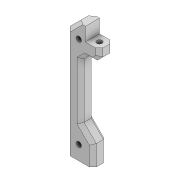
# Autodesk Inventor part: rackstand-v2-left
Saved by Autodesk Inventor 2020 (Build 240168000, 168)
## iProperties
Created: 2021-07-06
Part Number: rackstand-v2-left
Material: Generic
Document SubType Name: Modeling
Designer: Aidan Lee
Density: 1 g/cm^3
Appearance: Default
Author: Aidan Lee
Autodesk Inventor part; units mm, degrees
ref_plane "YZ Plane" through (0, 0, 0) normal (1, 0, 0) x (0, 1, 0)
sketch "Sketch1" plane through (0, 0, 0) normal (0, 0, 1) x (1, 0, 0)
  line L0 (37.5, 112.2656) -> (37.5, -3.3598) construction
  line L1 (37.5, 136.6711) -> (12.8431, 136.6711)
  line L2 (12.8431, 136.6711) -> (3.4308, 127.2588)
  line L3 (21.5, 136.6711) -> (21.5, 121.1711)
  line L4 (21.5, 121.1711) -> (37.5, 121.1711)
  line L5 (7.5005, 125.6717) -> (18.5, 136.6711) construction
  circle A0 centre (74.25, 61.25) radius 56.25 construction
  line L6 (37.5, 121.1711) -> (111, 121.1711) construction
  line L7 (111, 121.1711) -> (111, 150.3493) construction
  line L8 (111, 150.3493) -> (37.5, 150.3493) construction
  line L9 (37.5, 150.3493) -> (37.5, 121.1711) construction
  line L10 (37.5, 112.2656) -> (31.2028, 105.9683)
  line L11 (31.2028, 105.9683) -> (22.2972, 105.9683)
  line L12 (22.2972, 105.9683) -> (16, 99.6711)
  line L13 (16, 99.6711) -> (16, 37.1221)
  line L14 (16, 37.1221) -> (30, 23.1221)
  line L15 (30, 23.1221) -> (30, 0)
  line L16 (30, 0) -> (0, 0)
  line L17 (0, 0) -> (0, 123.828)
  line L18 (3.4308, 127.2588) -> (0, 123.828)
  line L19 (18, 73.8677) -> (18, 48.6323) construction
  line L20 (83.3625, 5) -> (65.1375, 5) construction
  line L21 (37.5, 121.1711) -> (37.5, 136.6711)
  line L22 (37.5, 121.1711) -> (37.5, 112.2656)
  line L23 (35.2471, 20.7034) -> (29.4259, 26.5246) construction
  point P0 (19.5296, 140.85)
  point P1 (74.25, 121.1711)
  point P2 (18, 61.25)
  point P3 (74.25, 5)
  dimension "d32" = 15.5
  dimension "d33" = 16
  dimension "d34" = 8.6569
  dimension "d38" = 4
  dimension "d39" = 3
  dimension "d65" = 112.5
  dimension "d66" = 70.293
  dimension "d67" = 73.5
  dimension "d70" = 45
  dimension "d71" = 16
  dimension "d72" = 2
  dimension "d73" = 5
  dimension "d74" = 30
  dimension "d75" = 2
  constraints: 48 end point, 7 parallel, 7 perpendicular, 4 horizontal, 3 equal length, 3 midpoint, 3 tangent, 3 vertical, 2 collinear, 2 point on circle, 2 point on line, 1 centre point, 1 coincident, 1 horizontal alignment, 1 vertical alignment
  measures "d32" distance of L3.start L3.end
  measures "d33" distance of L3.end L4.end
  measures "d34" distance from line of L1.end L3
  measures "d38" distance between parallel lines of L5 L2
  measures "d39" distance from line of L5.end L3
  measures "d65" diameter of A0
  measures "d66" distance of L4.end A0.centre
  measures "d67" distance of L7.end L8.end
  measures "d70" angle of L1 L2
  measures "d71" distance between parallel lines of L17 L13
  measures "d72" distance between parallel lines of L19 L13
  measures "d73" distance from line of L15.end L20
  measures "d74" distance between parallel lines of L17 L15
  measures "d75" distance between parallel lines of L14 L23
extrude "Extrusion2" add sketch "Sketch1" along normal blind 16 contours L3 L4 L22 L10 L11 L12 L13 L14 L15 L16 L17 L18 L2 L1
ref_plane "Work Plane3" through (21.5, 121.1711, 16) normal (0, 1, 0) x (1, 0, 0)
sketch "Sketch4" plane through (21.5, 121.1711, 16) normal (0, 1, 0) x (1, 0, 0)
  circle A0 centre (8, 8) radius 3
  line L0 (16, 16) -> (0, 16) projected
  line L1 (16, 16) -> (16, 0) projected
  point P0 (-21.5, 16)
  point P1 (16, 8)
  point P2 (8, 16)
  dimension "d76" = 6
  constraints: 2 midpoint, 1 centre point, 1 horizontal alignment, 1 vertical alignment
  measures "d76" diameter of A0
hole "Hole1" at (29.5, 121.1711, 8) direction (0, -1, 0) diameter 6 depth 9.5 tip angle 118
ref_plane "Work Plane2" through (4, 0, 0) normal (0, -1, 0) x (1, 0, 0)
sketch "Sketch5" plane through (4, 0, 0) normal (0, -1, 0) x (1, 0, 0)
  circle A0 centre (3.5, 8) radius 3
  line L0 (11, 48.9313) -> (11, 41.3239)
  circle A1 centre (18.5, 8) radius 3
  line L1 (-4, 0) -> (26, 0) projected
  line L2 (26, 0) -> (26, 16) projected
  point P0 (11, 0)
  point P1 (26, 8)
  dimension "d52" = 6
  dimension "d77" = 15
  constraints: 2 centre point, 2 end point, 2 midpoint, 1 horizontal alignment, 1 symmetric about line, 1 vertical, 1 vertical alignment, 1 other
  measures "d52" diameter of A0
  measures "d77" distance of A1.centre A0.centre
hole "Hole2" at (7.5, 0, 8) at (22.5, 0, 8) direction (0, 1, 0) diameter 6 depth 15 tip angle 118
thread "Thread4" size "M6x1" class "6H" standard "ANSI Metric M Profile" full length
thread "Thread5" size "M6x1" class "6H" standard "ANSI Metric M Profile" full length
chamfer "Chamfer2" distance 4 angle 45 18 edges at (0, 61.914, 16) (6.4216, 130.2496, 16) (6.4216, 130.2496, 0) (0, 61.914, 0) (34.3514, 109.1169, 0) (26.75, 105.9683, 0) (19.1486, 102.8197, 0) (16, 68.3966, 0) (23, 30.1221, 0) (30, 11.561, 0) (34.3514, 109.1169, 16) (26.75, 105.9683, 16) (19.1486, 102.8197, 16) (16, 68.3966, 16) (23, 30.1221, 16) (30, 11.561, 16) (37.5, 116.7183, 16) (37.5, 116.7183, 0)
sketch "Sketch6" plane through (0, 0, 16) normal (0, 0, 1) x (1, 0, 0)
  circle A0 centre (14.1, 120.25) radius 3
  circle A1 centre (14.1, 16.25) radius 3
  line L0 (4, 0) -> (4, 122.1711) projected
  circle A2 centre (74.25, 61.25) radius 56.25 construction
  circle A3 centre (74.25, 61.25) radius 50 construction
  line L1 (74.25, 111.25) -> (10.3895, 111.25) construction
  line L2 (0, 0) -> (4, 0) projected
  dimension "d88" = 100
  dimension "d85" = 6
  dimension "d86" = 10.1
  dimension "d89" = 9
  dimension "d103" = 104
  constraints: 2 centre point, 2 end point, 2 horizontal, 2 vertical alignment, 1 coincident, 1 equal radius, 2 other
  measures "d85" diameter of A0
  measures "d86" distance from line of L0 A0.centre
  measures "d89" distance from line of L1 A0.centre
  measures "d103" distance of A0.centre A1.centre
hole "Hole3" at (14.1, 120.25, 16) at (14.1, 16.25, 16) direction (0, 0, -1) diameter 6 depth 10 tip angle 118
thread "Thread8" size "M6x1" class "6H" standard "ANSI Metric M Profile" full length
thread "Thread9" size "M6x1" class "6H" standard "ANSI Metric M Profile" full length
body "Solid2"
